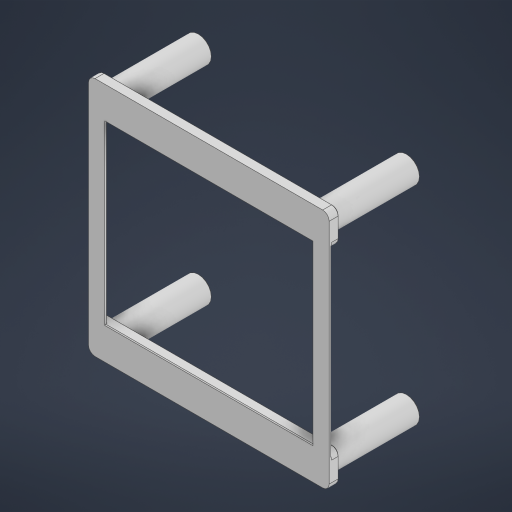
# Autodesk Inventor part: ScanCoverMount
Saved by Autodesk Inventor 2023 (Build 270158000, 158)
## iProperties
Created: 2023-12-11
Part Number: ScanCoverMount
Material: Generic
Document SubType Name: Modeling
Designer: FizzyApple12
Density: 1 g/cm^3
Appearance: Default
Author: FizzyApple12
Autodesk Inventor part; units mm, degrees
ref_plane "YZ Plane" through (0, 0, 0) normal (1, 0, 0) x (0, 1, 0)
ref_plane "XZ Plane" through (0, 0, 0) normal (0, 1, 0) x (-1, 0, 0)
ref_plane "XY Plane" through (0, 0, 0) normal (0, 0, 1) x (1, 0, 0)
sketch "Sketch1" plane through (0, 0, 0) normal (0, 0, 1) x (1, 0, 0)
  line L0 (0, 0) -> (-74, 0)
  line L1 (-74, 0) -> (-74, 10)
  line L2 (-74, 10) -> (0, 10)
  line L3 (0, 10) -> (0, 0)
  line L4 (-74, 10) -> (-64, 0) construction
  line L5 (0, 10) -> (-10, 0) construction
  circle A0 centre (-69, 5) radius 4
  circle A1 centre (-5, 5) radius 4
  circle A2 centre (-69, 5) radius 1.45
  circle A3 centre (-5, 5) radius 1.45
  line L6 (0, -64) -> (-74, -64)
  line L7 (-74, -64) -> (-74, -54)
  line L8 (-74, -54) -> (0, -54)
  line L9 (0, -54) -> (0, -64)
  line L10 (-74, -54) -> (-64, -64) construction
  line L11 (0, -54) -> (-10, -64) construction
  circle A4 centre (-69, -59) radius 4
  circle A5 centre (-5, -59) radius 4
  circle A6 centre (-69, -59) radius 1.45
  circle A7 centre (-5, -59) radius 1.45
  line L12 (-74, -54) -> (-69, -54)
  line L13 (-69, -54) -> (-69, 0)
  line L14 (-69, 0) -> (-74, 0)
  line L15 (-74, 0) -> (-74, -54)
  line L16 (0, -54) -> (-5, -54)
  line L17 (-5, -54) -> (-5, 0)
  line L18 (-5, 0) -> (0, 0)
  line L19 (0, 0) -> (0, -54)
  point P0 (-5, 0)
  point P1 (-69, -54)
  dimension "d0" = 74
  dimension "d1" = 10
  dimension "d2" = 45
  dimension "d3" = 8
  dimension "d5" = 2.9
  dimension "d22" = 74
  dimension "d23" = 5
  constraints: 40 end point, 8 centre point, 8 parallel, 6 equal radius, 5 equal length, 5 point on line, 4 coincident, 4 horizontal, 4 midpoint, 4 perpendicular, 2 collinear
  measures "d0" distance of L1.end L2.end
  measures "d1" distance of L0.end L1.end
  measures "d2" angle of L2 L4
  measures "d3" diameter of A0
  measures "d5" diameter of A2
  measures "d22" distance between parallel lines of L2 L6
  measures "d23" distance between parallel lines of L15 L13
extrude "Extrusion1" add sketch "Sketch1" against normal blind 3 contours L0 L1 L2 L3 | L9 L6 L7 L8 | A0 | A1 | A2 | A3 | A4 | A5 | A6 | A7
extrude "Extrusion2" add sketch "Sketch1" against normal blind 29 contours A0 | A1 | A4 | A5
extrude "Extrusion3" add sketch "Sketch1" against normal blind 0.5 contours L19 L8 L17 L0 | L13 L8 L15 L0
fillet "Fillet1" radius 2 8 edges at (-74, 10, -1.5) (-74, 0, -1.75) (0, 10, -1.5) (0, 0, -1.75) (-74, -54, -1.75) (-74, -64, -1.5) (0, -54, -1.75) (0, -64, -1.5)
chamfer "Chamfer1" distance 0.25 angle 45 34 edges at (-37, 10, -3) (-0.5858, 9.4142, -3) (0, 5, -3) (-0.5858, 0.5858, -3) (-37, 0, -3) (-73.4142, 0.5858, -3) (-74, 5, -3) (-73.4142, 9.4142, -3) (-37, 0, 0) (-9, 5, -29) (-6.45, 5, -29) (-73, 5, -29) (-70.45, 5, -29) (-37, -54, -3) (-0.5858, -54.5858, -3) (0, -59, -3) (-0.5858, -63.4142, -3) (-37, -64, -3) (-73.4142, -63.4142, -3) (-74, -59, -3) (-73.4142, -54.5858, -3) (-37, -54, 0) (-73, -59, -29) (-70.45, -59, -29) (-9, -59, -29) (-6.45, -59, -29) (-70.5, 0, -0.5) (-3.5, 0, -0.5) (-3.5, -54, -0.5) (-70.5, -54, -0.5) (-6.45, -59, -3) (-6.45, 5, -3) (-70.45, 5, -3) (-70.45, -59, -3)
body "Solid1"
